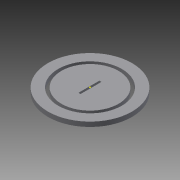
# Autodesk Inventor part: InnerCup
Saved by Autodesk Inventor 2015 (Build 190159000, 159)
## iProperties
Created: 2015-02-13
Part Number: InnerCup
Material: Generic
Document SubType Name: Modeling
Designer: Qiuyang
Density: 1 g/cm^3
Appearance: Default
Author: Qiuyang
Autodesk Inventor part; units mm, degrees
ref_plane "YZ Plane" through (0, 0, 0) normal (1, 0, 0) x (0, 1, 0)
ref_plane "XZ Plane" through (0, 0, 0) normal (0, 1, 0) x (-1, 0, 0)
ref_plane "XY Plane" through (0, 0, 0) normal (0, 0, 1) x (1, 0, 0)
sketch "Sketch1" plane through (0, 0, 0) normal (0, 1, 0) x (-1, 0, 0)
  circle A0 centre (0, 0) radius 34.544
  circle A1 centre (0, 0) radius 38.481
  circle A2 centre (0, 0) radius 50.8
  line L0 (1.27, 12.7) -> (-1.27, 12.7)
  line L1 (-1.27, 12.7) -> (-1.27, -12.7)
  line L2 (-1.27, -12.7) -> (1.27, -12.7)
  line L3 (1.27, -12.7) -> (1.27, 12.7)
  dimension "d0" = 69.088
  dimension "d1" = 76.962
  dimension "d2" = 101.6
  dimension "d6" = 2.54
  dimension "d7" = 25.4
  constraints: 8 end point, 3 centre point, 3 coincident, 2 parallel, 1 horizontal, 1 perpendicular
  measures "d0" diameter of A0
  measures "d1" diameter of A1
  measures "d2" diameter of A2
  measures "d6" distance of L2.end L1.end
  measures "d7" distance of L1.end L0.end
extrude "Extrusion1" add sketch "Sketch1" along normal blind 5.588 contours A0 | A2 | L3 L2 L1 L0
sketch "Sketch2" plane through (0, 5.588, 0) normal (0, 1, 0) x (1, 0, 0)
  line L0 (1.27, 12.7) -> (-1.27, 12.7)
  line L1 (-1.27, 12.7) -> (-1.27, -12.7)
  line L2 (-1.27, -12.7) -> (1.27, -12.7)
  line L3 (1.27, -12.7) -> (1.27, 12.7)
  point P0 (0, 0)
  dimension "d8" = 2.54
  dimension "d9" = 25.4
  constraints: 8 end point, 2 parallel, 1 horizontal, 1 perpendicular
  measures "d8" distance of L2.end L1.end
  measures "d9" distance of L1.end L0.end
extrude "Extrusion2" cut sketch "Sketch2" against normal blind 5.588
sketch "Sketch3" plane through (0, 5.588, 0) normal (0, 1, 0) x (1, 0, 0)
  point P0 (0, 0)
body "Solid1"
